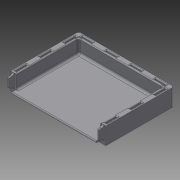
# Autodesk Inventor part: base_bottomrotateBox
Saved by Autodesk Inventor 2014 (Build 180170000, 170)
## iProperties
Created: 2014-04-22
Part Number: base_bottomrotateBox
Material: Generic
Document SubType Name: Modeling
Designer: t_emanb
Density: 1 g/cm^3
Appearance: Default
Author: t_emanb
Autodesk Inventor part; units mm, degrees
ref_plane "YZ Plane" through (0, 0, 0) normal (1, 0, 0) x (0, 1, 0)
ref_plane "XZ Plane" through (0, 0, 0) normal (0, 1, 0) x (-1, 0, 0)
ref_plane "XY Plane" through (0, 0, 0) normal (0, 0, 1) x (1, 0, 0)
sketch "Sketch1" plane through (0, 0, 0) normal (0, 1, 0) x (-1, 0, 0)
  line L0 (0, 0) -> (133.35, 0)
  line L1 (133.35, 0) -> (133.35, 95.25)
  line L2 (133.35, 95.25) -> (0, 95.25)
  line L3 (0, 95.25) -> (0, 0)
  dimension "d0" = 133.35
  dimension "d1" = 95.25
  constraints: 8 end point, 2 parallel, 1 horizontal, 1 perpendicular
  measures "d0" distance of L0.start L0.end
  measures "d1" distance of L2.end L0.start
extrude "Extrusion1" add sketch "Sketch1" along normal blind 5.08
sketch "Sketch2" plane through (0, 5.08, 0) normal (0, 1, 0) x (1, 0, 0)
  line L0 (0, 0) -> (-133.35, 0) projected
  line L1 (-133.35, 0) -> (-133.35, -95.25) projected
  line L2 (-133.35, -95.25) -> (0, -95.25) projected
  line L3 (0, -95.25) -> (0, 0) projected
  line L4 (-125.73, -7.62) -> (-7.62, -7.62)
  line L5 (-7.62, -7.62) -> (-7.62, -95.25)
  line L6 (-125.73, -95.25) -> (-125.73, -7.62)
  dimension "d4" = 7.62
  dimension "d5" = 7.62
  dimension "d6" = 7.62
  constraints: 6 end point, 2 point on line
  measures "d4" distance between parallel lines of L1 L6
  measures "d5" distance between parallel lines of L3 L5
  measures "d6" distance between parallel lines of L0 L4
extrude "Extrusion2" add sketch "Sketch2" along normal blind 19.05 contours L3 L2 L5 L4 L6 L1 L0
sketch "Sketch3" plane through (0, 24.13, 0) normal (0, 1, 0) x (1, 0, 0)
  line L0 (0, 0) -> (-133.35, 0) projected
  line L1 (-133.35, 0) -> (-133.35, -95.25) projected
  line L2 (-125.73, -95.25) -> (-125.73, -7.62) projected
  line L3 (-125.73, -7.62) -> (-7.62, -7.62) projected
  line L4 (-125.73, -2.54) -> (-110.49, -2.54)
  line L5 (-110.49, -2.54) -> (-110.49, -5.08)
  line L6 (-110.49, -5.08) -> (-125.73, -5.08)
  line L7 (-125.73, -5.08) -> (-125.73, -2.54)
  line L8 (-130.81, -7.62) -> (-128.27, -7.62)
  line L9 (-128.27, -7.62) -> (-128.27, -22.86)
  line L10 (-128.27, -22.86) -> (-130.81, -22.86)
  line L11 (-130.81, -22.86) -> (-130.81, -7.62)
  line L12 (-91.44, -2.54) -> (-76.2, -2.54)
  line L13 (-76.2, -2.54) -> (-76.2, -5.08)
  line L14 (-76.2, -5.08) -> (-91.44, -5.08)
  line L15 (-91.44, -5.08) -> (-91.44, -2.54)
  line L16 (-57.15, -2.54) -> (-41.91, -2.54)
  line L17 (-41.91, -2.54) -> (-41.91, -5.08)
  line L18 (-41.91, -5.08) -> (-57.15, -5.08)
  line L19 (-57.15, -5.08) -> (-57.15, -2.54)
  line L20 (-22.86, -2.54) -> (-7.62, -2.54)
  line L21 (-7.62, -2.54) -> (-7.62, -5.08)
  line L22 (-7.62, -5.08) -> (-22.86, -5.08)
  line L23 (-22.86, -5.08) -> (-22.86, -2.54)
  line L24 (-130.81, -41.91) -> (-128.27, -41.91)
  line L25 (-128.27, -41.91) -> (-128.27, -57.15)
  line L26 (-128.27, -57.15) -> (-130.81, -57.15)
  line L27 (-130.81, -57.15) -> (-130.81, -41.91)
  line L28 (-130.81, -76.2) -> (-128.27, -76.2)
  line L29 (-128.27, -76.2) -> (-128.27, -91.44)
  line L30 (-128.27, -91.44) -> (-130.81, -91.44)
  line L31 (-130.81, -91.44) -> (-130.81, -76.2)
  line L32 (-66.675, 0) -> (-66.675, -95.25) construction
  line L33 (-2.54, -7.62) -> (-5.08, -7.62)
  line L34 (-5.08, -7.62) -> (-5.08, -22.86)
  line L35 (-5.08, -22.86) -> (-2.54, -22.86)
  line L36 (-2.54, -22.86) -> (-2.54, -7.62)
  line L37 (-2.54, -41.91) -> (-5.08, -41.91)
  line L38 (-5.08, -41.91) -> (-5.08, -57.15)
  line L39 (-5.08, -57.15) -> (-2.54, -57.15)
  line L40 (-2.54, -57.15) -> (-2.54, -41.91)
  line L41 (-2.54, -76.2) -> (-5.08, -76.2)
  line L42 (-5.08, -76.2) -> (-5.08, -91.44)
  line L43 (-5.08, -91.44) -> (-2.54, -91.44)
  line L44 (-2.54, -91.44) -> (-2.54, -76.2)
  dimension "d9" = 15.24
  dimension "d10" = 15.24
  dimension "d11" = 2.54
  dimension "d12" = 2.54
  dimension "d13" = 2.54
  dimension "d14" = 2.54
  dimension "d17" = 34.29
  dimension "d24" = 34.29
  constraints: 82 end point, 12 symmetric about line, 5 parallel, 3 horizontal, 2 collinear, 2 perpendicular, 1 midpoint, 1 vertical, 40 other
  measures "d9" distance of L4.start L4.end
  measures "d10" distance of L10.end L8.start
  measures "d11" distance of L6.end L4.start
  measures "d12" distance of L8.start L8.end
  measures "d13" distance between parallel lines of L3 L6
  measures "d14" distance between parallel lines of L1 L11
  measures "d17" distance of L4.end L12.end
  measures "d24" distance of L8.start L24.start
extrude "Extrusion3" cut sketch "Sketch3" against normal blind 8.89
sketch "Sketch4" plane through (-133.35, 0, 95.25) normal (0, 0, 1) x (1, 0, 0)
  line L0 (0, 0) -> (133.35, 0) projected
  line L1 (7.62, 5.08) -> (125.73, 5.08) projected
  line L2 (0, 24.13) -> (7.62, 24.13) projected
  line L3 (0, 0) -> (0, 24.13) projected
  line L4 (2.54, 21.59) -> (5.08, 21.59)
  line L5 (5.08, 21.59) -> (5.08, 7.62)
  line L6 (5.08, 7.62) -> (2.54, 7.62)
  line L7 (2.54, 7.62) -> (2.54, 21.59)
  line L8 (7.62, 5.08) -> (7.62, 2.54)
  line L9 (7.62, 2.54) -> (125.73, 2.54)
  line L10 (125.73, 2.54) -> (125.73, 5.08)
  line L11 (66.675, 0) -> (66.675, 19.05) construction
  line L12 (130.81, 21.59) -> (128.27, 21.59)
  line L13 (128.27, 21.59) -> (128.27, 7.62)
  line L14 (128.27, 7.62) -> (130.81, 7.62)
  line L15 (130.81, 7.62) -> (130.81, 21.59)
  dimension "d31" = 2.54
  dimension "d32" = 2.54
  dimension "d33" = 2.54
  dimension "d34" = 2.54
  dimension "d35" = 13.97
  constraints: 24 end point, 5 parallel, 4 symmetric about line, 2 perpendicular, 1 horizontal, 1 midpoint
  measures "d31" distance between parallel lines of L1 L9
  measures "d32" distance of L4.start L4.end
  measures "d33" distance between parallel lines of L3 L7
  measures "d34" distance between parallel lines of L2 L4
  measures "d35" distance of L6.end L4.start
extrude "Extrusion4" add sketch "Sketch4" along normal blind 6.35
fillet "Fillet1" radius 3.175 7 edges at (0, 12.065, 0) (-133.35, 12.065, 0) (-125.73, 5.08, 51.435) (-66.675, 5.08, 7.62) (-7.62, 5.08, 51.435) (-7.62, 14.605, 7.62) (-125.73, 14.605, 7.62)
fillet "Fillet3" radius 3.175 4 edges at (-129.54, 7.62, 95.25) (-3.81, 7.62, 95.25) (-129.54, 21.59, 95.25) (-3.81, 21.59, 95.25)
fillet "Fillet4" radius 2.54 20 edges at (-129.54, 15.24, 91.44) (-129.54, 15.24, 76.2) (-129.54, 15.24, 41.91) (-129.54, 15.24, 57.15) (-129.54, 15.24, 22.86) (-129.54, 15.24, 7.62) (-110.49, 15.24, 3.81) (-125.73, 15.24, 3.81) (-91.44, 15.24, 3.81) (-76.2, 15.24, 3.81) (-57.15, 15.24, 3.81) (-41.91, 15.24, 3.81) (-22.86, 15.24, 3.81) (-7.62, 15.24, 3.81) (-3.81, 15.24, 22.86) (-3.81, 15.24, 7.62) (-3.81, 15.24, 57.15) (-3.81, 15.24, 41.91) (-3.81, 15.24, 76.2) (-3.81, 15.24, 91.44)
fillet "Fillet5" radius 1.27 7 edges at (-66.675, 2.54, 95.25) (-66.675, 2.54, 101.6) (-66.675, 5.08, 101.6) (-129.54, 7.62, 101.6) (-129.54, 21.59, 101.6) (-3.81, 7.62, 101.6) (-3.81, 21.59, 101.6)
fillet "Fillet6" radius 1.27 45 edges at (-130.81, 24.13, 83.82) (-129.54, 24.13, 76.2) (-128.27, 24.13, 83.82) (-129.54, 24.13, 91.44) (-130.81, 24.13, 49.53) (-129.54, 24.13, 41.91) (-128.27, 24.13, 49.53) (-129.54, 24.13, 57.15) (-130.81, 24.13, 15.24) (-129.54, 24.13, 7.62) (-128.27, 24.13, 15.24) (-129.54, 24.13, 22.86) (-125.73, 24.13, 3.81) (-118.11, 24.13, 2.54) (-110.49, 24.13, 3.81) (-118.11, 24.13, 5.08) (-91.44, 24.13, 3.81) (-83.82, 24.13, 2.54) (-76.2, 24.13, 3.81) (-83.82, 24.13, 5.08) (-57.15, 24.13, 3.81) (-49.53, 24.13, 2.54) (-41.91, 24.13, 3.81) (-49.53, 24.13, 5.08) (-22.86, 24.13, 3.81) (-15.24, 24.13, 2.54) (-7.62, 24.13, 3.81) (-15.24, 24.13, 5.08) (-3.81, 24.13, 22.86) (-5.08, 24.13, 15.24) (-3.81, 24.13, 7.62) (-2.54, 24.13, 15.24) (-5.08, 24.13, 49.53) (-3.81, 24.13, 41.91) (-2.54, 24.13, 49.53) (-3.81, 24.13, 57.15) (-5.08, 24.13, 83.82) (-3.81, 24.13, 76.2) (-2.54, 24.13, 83.82) (-3.81, 24.13, 91.44) (-124.8001, 24.13, 8.5499) (-66.675, 24.13, 7.62) (-8.5499, 24.13, 8.5499) (-7.62, 24.13, 53.0225) (-125.73, 24.13, 53.0225)
equation "\"d5\" = d4"
equation "\"d6\" = d4"
equation "\"d10\" = d9"
equation "\"d12\" = d11"
equation "\"d14\" = d13"
body "Solid1"
